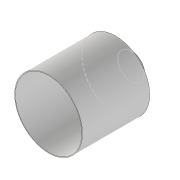
# Autodesk Inventor part: Tank_1
Saved by Autodesk Inventor 2020 (Build 240168000, 168)
## iProperties
Created: 2020-04-08
Part Number: Tank_1
Material: Generisch
Document SubType Name: Modeling
Designer: franz
Density: 1 g/cm^3
Appearance: Vorgabe
Author: franz
Autodesk Inventor part; units mm, degrees
ref_plane "YZ Plane" through (0, 0, 0) normal (1, 0, 0) x (0, 1, 0)
ref_plane "XZ Plane" through (0, 0, 0) normal (0, 1, 0) x (-1, 0, 0)
ref_plane "XY Plane" through (0, 0, 0) normal (0, 0, 1) x (1, 0, 0)
sketch "Skizze1" plane through (0, 0, 0) normal (0, 1, 0) x (-1, 0, 0)
  line L0 (0, 82.3152) -> (0, -45.1122)
  line L1 (250, 500) -> (250, 0)
  line L2 (250, 0) -> (250, 0)
  line L3 (250, 0) -> (100, -116.2752)
  line L4 (100, -116.2752) -> (100, -122.6015)
  line L5 (100, -122.6015) -> (251.711, -5)
  line L6 (251.711, -5) -> (255, -5)
  line L7 (255, -5) -> (255, 500)
  line L8 (255, 500) -> (250, 500)
  line L9 (306, 0) -> (-51, 0) projected
  point P0 (0, 0)
  dimension "d0" = 5
  dimension "d1" = 5
  dimension "d2" = 5
  dimension "d3" = 500
  dimension "d4" = 500
  dimension "d5" = 500
  dimension "d6" = 200
  constraints: 18 end point, 4 parallel, 3 vertical, 2 perpendicular, 1 collinear
  measures "d0" distance between parallel lines of L7 L1
  measures "d1" distance between parallel lines of L6 L2
  measures "d2" distance between parallel lines of L5 L3
  measures "d3" diameter of L1 L0
  measures "d4" distance of L1.start L1.end
  measures "d5" diameter of L2.end L0
  measures "d6" diameter of L4 L0
revolve "Umdrehung1" add sketch "Skizze1" angle 360 about axis through (0, 0, 82.3152) along (0, 0, -1)
sketch "Skizze3" plane through (0, 0, 0) normal (0, 1, 0) x (-1, 0, 0)
  line L0 (-251.711, -5) -> (-100, -122.6015) projected
  line L1 (-397.6603, 108.1352) -> (-63.9838, -150.52)
  point P0 (0, 0)
  constraints: 2 end point, 1 collinear
ref_plane "Arbeitsebene1" through (397.6603, 0, 108.1352) normal (-0.6127, 0, 0.7904) x (0, -1, 0)
sketch "Skizze4" plane through (397.6603, 0, 108.1352) normal (-0.6127, 0, 0.7904) x (0, -1, 0)
  circle A0 centre (0, -278.6039) radius 90
  ellipse E0 centre (0, -383.6039) end of major axis (251.711, -383.6039) minor radius 198.94 projected
  point P0 (0, -380.5407)
  dimension "d12" = 180
  dimension "d13" = 105
  constraints: 1 centre point
  measures "d12" diameter of A0
  measures "d13" distance of E0.centre A0.centre
extrude "Extrusion2" add sketch "Skizze4" along normal up to surface contours A0
sketch "Skizze5" plane through (397.6603, 0, 108.1352) normal (0.6127, 0, -0.7904) x (-0.7904, 0, -0.6127)
  circle A0 centre (278.6039, 0) radius 85
  arc A1 (368.6039, 0) -> (188.6039, 0) centre (278.6039, 0) ccw projected
  point P0 (380.5407, 0)
  dimension "d16" = 170
  constraints: 1 centre point, 1 coincident
  measures "d16" diameter of A0
extrude "Extrusion3" cut sketch "Skizze5" against normal up to surface
equation "\"d1\" = d0"
equation "\"d2\" = d0"
